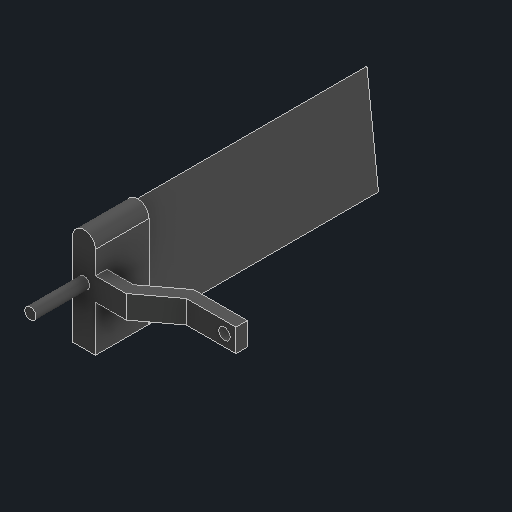
# Autodesk Inventor part: rudder_fin
Saved by Autodesk Inventor 2022.2 (Build 262287010, 287A)
## iProperties
Created: 2022-03-30
Part Number: rudder_fin
Material: Generic
Document SubType Name: Modeling
Designer: kardo
Density: 1 g/cm^3
Appearance: Dark Plastic
Author: kardo
Autodesk Inventor part; units mm, degrees
ref_plane "YZ Plane" through (0, 0, 0) normal (1, 0, 0) x (0, 1, 0)
ref_plane "XY Plane" through (0, 0, 0) normal (0, 0, 1) x (1, 0, 0)
derived "parameters_powertrain.ipt"
derived "rudder_base.ipt"
sketch "sk_base" plane through (0, 0, 0) normal (0, 1, 0) x (-1, 0, 0)
  line L0 (13.09, 0) -> (-13.09, 0) construction
  line L1 (0, -3.74) -> (0, 22.44) construction
  point P0 (0, 0)
  point P1 (0, 15.7)
  point P2 (0, 3)
  point P3 (0, 18.7)
sketch "sk_length" plane through (0, 0, 0) normal (0, 0, 1) x (1, 0, 0)
  line L0 (0, -62.4) -> (0, 10.4) construction
  line L1 (-5.6, 0) -> (5.6, 0) construction
  arc A0 (-2, -50) -> (2, -50) centre (0, -50) ccw
  line L2 (-2, -50) -> (-2, -40)
  line L3 (-2, -40) -> (2, -40)
  line L4 (2, -40) -> (2, -2)
  line L5 (2, -2) -> (-4, -2)
  line L6 (-4, -2) -> (-4, 0)
  line L7 (4, 0) -> (4, -46)
  line L8 (-4, 0) -> (4, 0)
  line L9 (2, -46) -> (2, -50)
  line L10 (4, -46) -> (2, -46)
  point P0 (0, 0)
sketch "Sketch3" plane through (0, 0, 0) normal (0, 0, 1) x (1, 0, 0)
  line L0 (-2, -40) -> (2, -40) construction
  arc A0 (2, -44) -> (-2, -44) centre (0, -44) ccw
  line L1 (-2, -44) -> (-2, -60)
  line L2 (2, -60) -> (2, -44)
  line L3 (-2, -60) -> (2, -60)
  point P0 (0, 0)
  point P1 (0, -50)
  dimension "d1" = 2
  dimension "d2" = 10
  constraints: 6 end point, 3 perpendicular, 2 point on circle, 2 point on line, 2 tangent, 1 centre point
  measures "d1" distance edge to line of A0 L0
  measures "d2" distance from line of L3 point (0, -50)
sketch "Sketch4" plane through (0, 0, 0) normal (0, 1, 0) x (-1, 0, 0)
  line L0 (0, 15.7) -> (0, 3)
  point P0 (0, 0)
  point P1 (0, 9.35)
  constraints: 2 end point, 1 midpoint
sketch "Sketch5" plane through (0, 0, 0) normal (0, 0, 1) x (1, 0, 0)
  arc A0 (2, -44) -> (-2, -44) centre (0, -44) ccw construction
  line L0 (-2, -60) -> (2, -60) projected
  line L1 (-2, -60) -> (0, -42)
  line L2 (2, -60) -> (0, -42)
  point P0 (0, 0)
  constraints: 4 end point, 1 point on circle
sketch "Sketch6" plane through (0, 0, 0) normal (0, 0, 1) x (1, 0, 0)
  circle A0 centre (0, -50) radius 1
  point P0 (0, 0)
  dimension "d7" = 2
  constraints: 1 centre point, 1 coincident
  measures "d7" diameter of A0
extrude "Extrusion1" add sketch "Sketch3" along normal up to surface (9.35 mm away)
extrude "Extrusion2" add sketch "Sketch5" against normal blind 40
extrude "Extrusion3" add sketch "Sketch6" along normal up to surface (18.7 mm away)
ref_plane "Work Plane1" through (0, -50, 0) normal (0, 1, 0) x (-1, 0, 0)
sketch "Sketch7" plane through (0, -50, 0) normal (0, 1, 0) x (-1, 0, 0)
  line L0 (0, -51.74) -> (0, 30.44) construction
  line L1 (8.2093, 0) -> (-21.2561, 0) construction
  line L2 (0, -90.65) -> (100, -90.65) construction
  line L3 (100, -90.65) -> (100, 0) construction
  line L4 (0, 15.7) -> (0, 3)
  line L5 (0, 9.35) -> (-7.3333, 9.35)
  line L6 (-7.3333, 9.35) -> (-13.3333, 4.85)
  line L7 (-13.3333, 4.85) -> (-20, 4.85)
  line L8 (-22, 4.85) -> (-22, 2.85)
  line L9 (-22, 2.85) -> (-12.6667, 2.85)
  line L10 (-12.6667, 2.85) -> (-6.6667, 7.35)
  line L11 (-6.6667, 7.35) -> (0, 7.35)
  line L12 (-6.6667, 7.35) -> (-13.3333, 7.35) construction
  line L13 (-13.3333, 7.35) -> (-13.3333, 4.85) construction
  line L14 (-20, 4.85) -> (-22, 4.85)
  point P0 (0, 0)
  dimension "d11" = 100
  dimension "d14" = 100
  dimension "d15" = 95.5
  dimension "d16" = 120
  dimension "d17" = 2
  dimension "d18" = 2
  dimension "d19" = 2
  dimension "d20" = 2
  constraints: 26 end point, 6 parallel, 3 perpendicular, 3 point on line, 2 collinear, 2 equal length, 1 midpoint
  measures "d11" distance between parallel lines of L3 L0
  measures "d14" distance from line of L2 L5.start
  measures "d15" distance from line of L2 L7.end
  measures "d16" distance from line of L7.end L3
  measures "d17" distance between parallel lines of L5 L11
  measures "d18" distance between parallel lines of L7 L9
  measures "d19" distance between parallel lines of L6 L10
  measures "d20" distance of L7.end L8.start
extrude "Extrusion4" add sketch "Sketch7" along normal mid plane 4
sketch "Sketch8" plane through (13.3333, -48, 4.85) normal (0, 0, 1) x (1, 0, 0)
  point P0 (-13.3333, 48)
  point P1 (6.6667, -2)
hole "Hole1" at (20, -50, 4.85) direction (0, 0, -1) diameter 2 end through all
equation "\"d15\" = d14 + rudder_joint_offset_vertical"
equation "\"d16\" = d11 + rudder_joint_offset_right"
equation "\"rudder_joint_offset_vertical\" = -4.5"
equation "\"rudder_joint_offset_right\" = 20"
body "Solid1"
